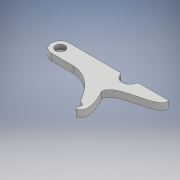
# Autodesk Inventor part: retreat
Saved by Autodesk Inventor 2018 (Build 220112000, 112)
## iProperties
Created: 2017-06-25
Part Number: retreat
Material: Generic
Document SubType Name: Modeling
Designer: theso
Density: 1 g/cm^3
Appearance: Default
Author: theso
Autodesk Inventor part; units mm, degrees
note: some values were not read from the file. Chosen so that the rebuilt part matches the saved one: edges of "Fillet2".
ref_plane "YZ Plane" through (0, 0, 0) normal (1, 0, 0) x (0, 1, 0)
ref_plane "XZ Plane" through (0, 0, 0) normal (0, 1, 0) x (-1, 0, 0)
ref_plane "XY Plane" through (0, 0, 0) normal (0, 0, 1) x (1, 0, 0)
sketch "Sketch1" plane through (0, 0, 0) normal (0, 0, 1) x (1, 0, 0)
  line L0 (15.7385, -0.0311) -> (-29.1749, -0.0311)
  line L1 (-29.1749, -0.0311) -> (2.0558, -0.0311) construction
  line L2 (-29.1749, -8.0311) -> (-19.1749, -8.0311)
  line L3 (-19.1749, -8.0311) -> (-9.0765, -8.6728) construction
  line L4 (-9.0765, -8.6728) -> (-1.6699, -24.4547) construction
  spline S0 degree 2 poles (-19.1749, -8.0311) (-9.0765, -8.6728) (-1.6699, -24.4547) knots 1 1 1 2 2 2
  line L5 (-1.6699, -24.4547) -> (2.9761, -22.4111) construction
  line L6 (2.9761, -22.4111) -> (-2.9231, -11.7108) construction
  spline S1 degree 2 poles (-1.6699, -24.4547) (2.9761, -22.4111) (-2.9231, -11.7108) knots 1 1 1 2 2 2
  line L7 (-2.9231, -11.7108) -> (-2.9231, -4.7242) construction
  line L8 (-2.9231, -4.7242) -> (18.0519, -6.1311) construction
  line L9 (18.0519, -6.1311) -> (15.7385, -0.0311) construction
  spline S2 degree 3 poles (-2.9231, -11.7108) (-2.9231, -4.7242) (18.0519, -6.1311) (15.7385, -0.0311) knots 1 1 1 1 2 2 2 2
  arc A0 (-29.1749, -0.0311) -> (-29.1749, -8.0311) centre (-29.1749, -4.0311) ccw
  circle A1 centre (-29.1749, -4.0311) radius 2.15
  point P0 (0, 0)
  dimension "d0" = 8
  dimension "d1" = 10
  dimension "d2" = 4.3
  constraints: 6 end point, 3 horizontal, 2 centre point, 2 point on circle, 1 coincident, 1 vertical, 9 other
  measures "d0" distance of L1.start L2.start
  measures "d1" distance of L2.start L3.start
  measures "d2" diameter of A1
extrude "Extrusion1" add sketch "Sketch1" along normal blind 3
sketch "Sketch2" plane through (0, 0, 3) normal (0, 0, 1) x (1, 0, 0)
  line L0 (15.7385, -0.0311) -> (-29.1749, -0.0311) projected
  line L1 (-29.1749, -0.0311) -> (-1.8249, -0.0311)
  circle A0 centre (-1.8249, -0.0311) radius 3.5
  point P0 (0, 0)
  dimension "d5" = 27.35
  dimension "d6" = 7
  constraints: 2 end point, 1 centre point, 1 coincident, 1 point on line
  measures "d5" distance of L0.end L1.end
  measures "d6" diameter of A0
extrude "Extrusion2" cut sketch "Sketch2" against normal blind 3
sketch "Sketch3" plane through (0, 0, 3) normal (0, 0, 1) x (1, 0, 0)
  line L0 (-1.6699, -24.4547) -> (-2.4199, -23.1557)
  line L1 (-1.6699, -24.4547) -> (-0.1699, -24.4547) construction
  line L2 (-3.7341, -20.8795) -> (-2.4199, -23.1557)
  line L3 (-2.4199, -23.1557) -> (-1.13, -22.0176) construction
  line L4 (-1.13, -22.0176) -> (-2.0449, -20.2761) construction
  line L5 (-2.0449, -20.2761) -> (-3.7341, -20.8795) construction
  spline S0 degree 3 poles (-2.4199, -23.1557) (-1.13, -22.0176) (-2.0449, -20.2761) (-3.7341, -20.8795) knots 1 1 1 1 2 2 2 2
  point P0 (0, 0)
  dimension "d9" = 1.5
  dimension "d10" = 120
  constraints: 6 end point, 1 equal length, 1 horizontal, 3 other
  measures "d9" distance of L0.start L0.end
  measures "d10" angle of L1 L0
extrude "Extrusion3" cut sketch "Sketch3" against normal blind 3
fillet "Fillet2" radius 2 1 edges at (-3.5248, -20.8155, 1.5)
chamfer "Chamfer1" distance 1.2 angle 45 1 edges at (-31.3249, -4.0311, 0)
fillet "Fillet4" radius 1 2 edges at (1.6751, -0.0311, 1.5) (-5.3249, -0.0311, 1.5)
body "Solid1"
